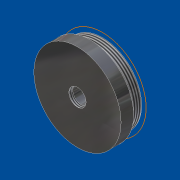
# Autodesk Inventor part: JF-AT-TC0007
Saved by Autodesk Inventor 2012 SP2 (Build 160219200, 219)
## iProperties
Created: 2010-03-15
Part Number: JF-AT-TC0007
Description: Botton Cap Air Tube
Document SubType Name: Modeling
Designer: S. Bassin
Density: 1.425 g/cm^3
Material: Acetal Resin, Black
Mass: 24.5473 g
Surface Area: 49.2388 cm^2
Volume: 17.2262 cm^3
Project: COMMON
Vendor: HHMI: JRC - ID&F
ALTERED ITEM PART NUMBER: N/A
ALTERED ITEM VENDOR: N/A
SPECIAL FINISH: NONE
SURFACE ROUGHNESS: N/A
LAB/DEPT: COMMON
REQUESTING SCIENTIST: COMMON
DESIGN DEPARTMENT: HHMI: JRC - ID&F
ALTERED ITEM DESCRIPTION: N/A
Author: S. Bassin
Revision Number: 0
Autodesk Inventor part; units mm, degrees
ref_plane "YZ Plane" through (0, 0, 0) normal (1, 0, 0) x (0, 1, 0)
ref_plane "XZ Plane" through (0, 0, 0) normal (0, 1, 0) x (-1, 0, 0)
ref_plane "XY Plane" through (0, 0, 0) normal (0, 0, 1) x (1, 0, 0)
sketch "Sketch1" plane through (0, 0, 0) normal (0, 0, 1) x (1, 0, 0)
  circle A0 centre (0, 0) radius 22.098
  dimension "d11" = 44.196
  constraints: 1 centre point, 1 coincident
  measures "d11" diameter of A0
extrude "Extrusion1" add sketch "Sketch1" along normal blind 12.7
sketch "Sketch2" plane through (0, 0, 12.7) normal (0, 0, 1) x (1, 0, 0)
  circle A0 centre (0, 0) radius 22.098 projected
  constraints: 1 coincident
hole "Hole1" at (0, 0, 12.7) direction (0, 0, -1) diameter 8.6106 depth 25.4 tip angle 118 thread size "1/8" designation "1/8 - 27 NPT" standard "NPT for PVC Pipe and Fitting"
sketch "Sketch3" plane through (0, 0, 0) normal (0, 0, -1) x (-1, 0, 0)
  circle A0 centre (0, 0) radius 4.3053 projected
  circle A1 centre (0, 0) radius 22.098 projected
sketch "Sketch4" plane through (0, 0, 0) normal (0, 0, -1) x (-1, 0, 0)
  circle A0 centre (0, 0) radius 22.098 projected
  circle A1 centre (0, 0) radius 19.8374
  dimension "d12" = 39.6748
  constraints: 1 centre point, 1 coincident
  measures "d12" diameter of A1
extrude "Extrusion2" cut sketch "Sketch4" against normal blind 6.35
thread "Thread1" size "1 9/16-20 UN" class "2A" standard "ANSI Unified Screw Threads" length 6.35
body "Solid1"
